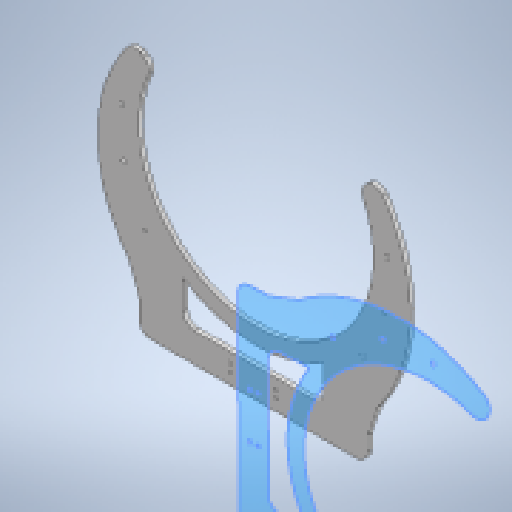
# Autodesk Inventor part: фанера_ухо
Saved by Autodesk Inventor 2023.1 (Build 271208000, 208)
## iProperties
Created: 2025-10-14
Part Number: фанера_ухо
Material: Типовые
Document SubType Name: Modeling
Designer: DELL
Density: 1 g/cm^3
Appearance: По умолчанию
Author: DELL
Autodesk Inventor part; units mm, degrees
ref_plane "YZ Plane" through (0, 0, 0) normal (1, 0, 0) x (0, 1, 0)
ref_plane "XZ Plane" through (0, 0, 0) normal (0, 1, 0) x (-1, 0, 0)
ref_plane "XY Plane" through (0, 0, 0) normal (0, 0, 1) x (1, 0, 0)
sketch "Эскиз1" plane through (0, 0, 0) normal (0, 0, 1) x (1, 0, 0)
  line L0 (12, 4) -> (40, 4) construction
  line L1 (0, 0) -> (52, 0) construction
  line L2 (-67.6811, -0.2343) -> (32.3189, -0.2343)
  line L3 (132.3189, 9.7657) -> (132.3189, 23.0512)
  line L4 (-77.6811, 26.4691) -> (-77.6811, 9.7657)
  line L5 (-77.6811, 26.4691) -> (-87.8723, 54.4691)
  line L6 (132.3189, 23.0512) -> (142.51, 51.0512)
  arc A0 (142.51, 51.0512) -> (146.8898, 221.5537) centre (23.3362, 139.42) ccw
  arc A1 (-90.1063, 221.3637) -> (-87.8723, 54.4691) centre (23.3362, 139.42) ccw
  arc A2 (-69.8234, 209.8708) -> (128.2861, 211.2859) centre (29.5436, 166.8699) ccw
  line L7 (-77.1442, 224.2501) -> (-74.1451, 222.5843)
  line L8 (133.7794, 224.7999) -> (132.6234, 224.1703)
  line L9 (-27.6811, 26.8699) -> (82.3189, 26.8699)
  line L10 (32.3189, -0.2343) -> (122.3189, -0.2343)
  line L11 (-37.6811, 36.8699) -> (-37.6811, 63.541)
  line L12 (92.3189, 36.8699) -> (92.3189, 60.779)
  arc A3 (-37.6811, 63.541) -> (92.3189, 60.779) centre (29.5436, 166.8699) ccw
  arc A4 (-37.6811, 36.8699) -> (-27.6811, 26.8699) centre (-27.6811, 36.8699) ccw
  arc A5 (82.3189, 26.8699) -> (92.3189, 36.8699) centre (82.3189, 36.8699) ccw
  arc A6 (-69.8234, 209.8708) -> (-74.1451, 222.5843) centre (-79.0009, 213.8423) ccw
  arc A7 (-77.1442, 224.2501) -> (-90.1063, 221.3637) centre (-82, 215.5082) ccw
  arc A8 (132.6234, 224.1703) -> (128.2861, 211.2859) centre (137.4059, 215.3881) ccw
  arc A9 (146.8898, 221.5537) -> (133.7794, 224.7999) centre (138.562, 216.0177) ccw
  circle A10 centre (5, 17) radius 1.6 projected
  circle A11 centre (5, 10) radius 1.6 projected
  circle A12 centre (47, 10) radius 1.6 projected
  circle A13 centre (47, 17) radius 1.6 projected
  arc A14 (-77.6811, 9.7657) -> (-67.6811, -0.2343) centre (-67.6811, 9.7657) ccw
  arc A15 (122.3189, -0.2343) -> (132.3189, 9.7657) centre (122.3189, 9.7657) ccw
  point P0 (-77.6811, -0.2343)
  point P1 (132.3189, -0.2343)
  point P2 (141.7652, 229.1487)
  point P3 (-65.8946, 218.0014)
  point P4 (26, 0)
  point P5 (77.3189, -0.2343)
  point P6 (-77.6811, 18.1174)
  point P7 (-37.6811, 50.2054)
  point P8 (132.3189, 16.4085)
  point P9 (92.3189, 48.8244)
  dimension "d21" = 167.1042
  dimension "d22" = 10
  dimension "d23" = 10
  dimension "d28" = 100
  dimension "d29" = 15
  dimension "d32" = 140
  dimension "d33" = 10
  dimension "d43" = 100
  dimension "d44" = 40
  dimension "d45" = 40
  dimension "d46" = 28
  dimension "d47" = 28
  dimension "d48" = 20
  dimension "d49" = 20
  constraints: 26 point on circle, 22 end point, 16 tangent, 12 centre point, 6 midpoint, 6 point on line, 5 equal radius, 5 perpendicular, 2 horizontal, 1 coincident, 1 parallel
  measures "d21" vertical distance of point (77.319, -0.234) A2.centre
  measures "d22" radius of A4
  measures "d23" radius of A6
  measures "d28" distance of L2.end point (132.319, -0.234)
  measures "d29" radial gap between concentric circles of A2 A3
  measures "d32" distance from line of L9 A3.centre
  measures "d33" radius of A14
  measures "d43" distance of L2.start L2.end
  measures "d44" horizontal distance of L4.start point (-37.681, 50.205)
  measures "d45" horizontal distance of point (132.319, 16.408) point (92.319, 48.824)
  measures "d46" vertical distance of L4.start L5.end
  measures "d47" vertical distance of L3.end L6.end
  measures "d48" angle of L3 L6
  measures "d49" angle of L4 L5
extrude "Выдавливание1" add sketch "Эскиз1" along normal blind 4
sketch "Эскиз2" plane through (0, 0, 4) normal (0, 0, 1) x (1, 0, 0)
  arc A0 (-77.1442, 224.2501) -> (-90.1063, 221.3637) centre (-82, 215.5082) ccw construction
  line L0 (-37.6811, 36.8699) -> (-37.6811, 63.541) construction
  arc A1 (-77.1442, 224.2501) -> (-37.6811, 50.2054) centre (34.7868, 158.1332) ccw construction
  circle A2 centre (-91.995, 129.3866) radius 2.1
  circle A3 centre (-72.2713, 84.3866) radius 2.1
  circle A4 centre (-94.1931, 174.3866) radius 2.1
  line L1 (-67.6811, -0.2343) -> (122.3189, -0.2343) construction
  circle A5 centre (5, 10) radius 1.6 construction
  circle A6 centre (47, 10) radius 1.6 construction
  line L2 (5, 10) -> (47, 10) construction
  line L3 (26, 10) -> (26, 211.5399) construction
  line L4 (92.3189, 60.779) -> (92.3189, 36.8699) projected
  arc A7 (132.6234, 224.1703) -> (128.2861, 211.2859) centre (137.4059, 215.3881) ccw projected
  arc A8 (92.3189, 48.8244) -> (132.6234, 224.1703) centre (21.0087, 157.5206) ccw construction
  line L5 (-72.2713, 84.3866) -> (128.4862, 84.3866) construction
  circle A9 centre (128.4862, 84.3866) radius 2.1
  line L6 (-91.995, 129.3866) -> (161.5686, 129.3866) construction
  circle A10 centre (147.9279, 129.3866) radius 2.1
  line L7 (-94.1931, 174.3866) -> (161.5686, 174.3866) construction
  circle A11 centre (149.91, 174.3866) radius 2.1
  point P0 (0, 0)
  dimension "d35" = 4.2
  dimension "d36" = 4.2
  dimension "d37" = 45
  dimension "d38" = 4.2
  dimension "d39" = 45
  dimension "d50" = 130
  dimension "d51" = 130
  dimension "d52" = 4.2
  dimension "d53" = 4.2
  dimension "d54" = 4.2
  constraints: 10 end point, 10 point on circle, 8 centre point, 4 horizontal, 3 midpoint, 2 point on line, 1 coincident, 1 vertical, 1 other
  measures "d35" diameter of A2
  measures "d36" diameter of A3
  measures "d37" vertical distance of L5.start L6.start
  measures "d38" diameter of A4
  measures "d39" vertical distance of L6.start L7.start
  measures "d50" radius of A8
  measures "d51" radius of A1
  measures "d52" diameter of A9
  measures "d53" diameter of A10
  measures "d54" diameter of A11
extrude "Выдавливание2" cut sketch "Эскиз2" against normal blind 4
